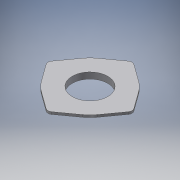
# Autodesk Inventor part: 付け根ロール_サブフレーム_1_3
Saved by Autodesk Inventor 2018 (Build 220112000, 112)
## iProperties
Created: 2016-05-02
Part Number: 付け根ロール_サブフレーム_1_3
Material: アルミニウム 2014-T4
Document SubType Name: Modeling
Designer: hiroaki
Density: 2.8 g/cm^3
Appearance: サテン
Mass: 6.12812 g
Surface Area: 34.4322 cm^2
Volume: 2.18861 cm^3
Author: hiroaki
Autodesk Inventor part; units mm, degrees
ref_plane "YZ Plane" through (0, 0, 0) normal (1, 0, 0) x (0, 1, 0)
ref_plane "XZ Plane" through (0, 0, 0) normal (0, 1, 0) x (-1, 0, 0)
ref_plane "XY Plane" through (0, 0, 0) normal (0, 0, 1) x (1, 0, 0)
derived "付け根ロール_基礎.ipt"
sketch "スケッチ1" plane through (0, 0, 0) normal (0, 0, 1) x (1, 0, 0)
  circle A0 centre (0, 0) radius 5.05 construction
  circle A1 centre (0, -8.5) radius 1.35 construction
  circle A2 centre (0, -8.5) radius 2.5 construction
  circle A3 centre (-5.6569, -5.6569) radius 1.55 construction
  line L0 (-5.6569, -5.6569) -> (0, 0) construction
  line L1 (0, 0) -> (0, -8.5) construction
  line L2 (-4.835, -8.7241) -> (-7.9022, -7.9022) construction
  line L3 (-7.9022, -7.9022) -> (-8.7241, -4.835) construction
  line L4 (-8.7241, -4.835) -> (-6.4787, -2.5896) construction
  line L5 (-6.4787, -2.5896) -> (-3.4115, -3.4115) construction
  line L6 (-3.4115, -3.4115) -> (-2.5896, -6.4787) construction
  line L7 (-2.5896, -6.4787) -> (-4.835, -8.7241) construction
  circle A4 centre (5.6569, -5.6569) radius 1.55 construction
  line L8 (8.7241, -4.835) -> (7.9022, -7.9022) construction
  line L9 (7.9022, -7.9022) -> (4.835, -8.7241) construction
  line L10 (4.835, -8.7241) -> (2.5896, -6.4787) construction
  line L11 (3.4115, -3.4115) -> (6.4787, -2.5896) construction
  line L12 (2.5896, -6.4787) -> (3.4115, -3.4115) construction
  line L13 (6.4787, -2.5896) -> (8.7241, -4.835) construction
  circle A5 centre (8.5, 0) radius 2.5 construction
  circle A6 centre (8.5, 0) radius 1.35 construction
  circle A7 centre (5.6569, 5.6569) radius 1.55 construction
  line L14 (4.835, 8.7241) -> (7.9022, 7.9022) construction
  line L15 (7.9022, 7.9022) -> (8.7241, 4.835) construction
  line L16 (8.7241, 4.835) -> (6.4787, 2.5896) construction
  line L17 (3.4115, 3.4115) -> (2.5896, 6.4787) construction
  line L18 (6.4787, 2.5896) -> (3.4115, 3.4115) construction
  line L19 (2.5896, 6.4787) -> (4.835, 8.7241) construction
  circle A8 centre (0, 8.5) radius 2.5 construction
  circle A9 centre (0, 8.5) radius 1.35 construction
  circle A10 centre (-5.6569, 5.6569) radius 1.55 construction
  line L20 (-8.7241, 4.835) -> (-7.9022, 7.9022) construction
  line L21 (-7.9022, 7.9022) -> (-4.835, 8.7241) construction
  line L22 (-4.835, 8.7241) -> (-2.5896, 6.4787) construction
  line L23 (-3.4115, 3.4115) -> (-6.4787, 2.5896) construction
  line L24 (-2.5896, 6.4787) -> (-3.4115, 3.4115) construction
  line L25 (-6.4787, 2.5896) -> (-8.7241, 4.835) construction
  circle A11 centre (-8.5, 0) radius 2.5 construction
  circle A12 centre (-8.5, 0) radius 1.35 construction
  circle A13 centre (0, 0) radius 12.45 construction
  circle A14 centre (0, 0) radius 21 construction
  circle A15 centre (0, 24.25) radius 3.25 construction
  circle A16 centre (0, 24.25) radius 1.05
  circle A17 centre (-24.25, 0) radius 1.05
  circle A18 centre (0, -24.25) radius 1.05
  circle A19 centre (24.25, 0) radius 1.05
  circle A20 centre (0, 0) radius 21.05 construction
  circle A21 centre (0, 0) radius 27.1368 construction
  circle A22 centre (0, 24.25) radius 2.8868 construction
  line L26 (2.5, 25.6934) -> (2.5, 22.8066) construction
  line L27 (2.5, 22.8066) -> (0, 21.3632) construction
  line L28 (0, 21.3632) -> (-2.5, 22.8066) construction
  line L29 (-2.5, 22.8066) -> (-2.5, 25.6934) construction
  line L30 (-2.5, 25.6934) -> (0, 27.1368) construction
  line L31 (0, 27.1368) -> (2.5, 25.6934) construction
  circle A23 centre (0, 0) radius 11.45
  circle A24 centre (0, 0) radius 22.55 construction
  arc A25 (-13.1973, 18.2848) -> (-18.2848, 13.1973) centre (0, 0) ccw
  line L32 (-13.1973, 18.2848) -> (-1.6895, 26.5907)
  arc A26 (1.6895, 26.5907) -> (-1.6895, 26.5907) centre (0, 24.25) ccw
  line L33 (1.6895, 26.5907) -> (13.1973, 18.2848)
  line L34 (0, 0) -> (0, 24.25) construction
  line L35 (0, 0) -> (8.5, 0) construction
  line L36 (-18.2848, 13.1973) -> (-26.5907, 1.6895)
  arc A27 (-26.5907, 1.6895) -> (-26.5907, -1.6895) centre (-24.25, 0) ccw
  line L37 (-26.5907, -1.6895) -> (-18.2848, -13.1973)
  arc A28 (-18.2848, -13.1973) -> (-13.1973, -18.2848) centre (0, 0) ccw
  line L38 (-13.1973, -18.2848) -> (-1.6895, -26.5907)
  arc A29 (-1.6895, -26.5907) -> (1.6895, -26.5907) centre (0, -24.25) ccw
  line L39 (1.6895, -26.5907) -> (13.1973, -18.2848)
  arc A30 (18.2848, 13.1973) -> (13.1973, 18.2848) centre (0, 0) ccw
  arc A31 (26.5907, -1.6895) -> (26.5907, 1.6895) centre (24.25, 0) ccw
  line L40 (26.5907, 1.6895) -> (18.2848, 13.1973)
  line L41 (26.5907, -1.6895) -> (18.2848, -13.1973)
  arc A32 (13.1973, -18.2848) -> (18.2848, -13.1973) centre (0, 0) ccw
  line L42 (2.75, 25.8377) -> (2.75, 22.6623)
  line L43 (2.75, 22.6623) -> (0, 21.0746)
  line L44 (0, 21.0746) -> (-2.75, 22.6623)
  line L45 (-2.75, 22.6623) -> (-2.75, 25.8377)
  line L46 (-2.75, 25.8377) -> (0, 27.4254)
  line L47 (0, 27.4254) -> (2.75, 25.8377)
  circle A33 centre (24.25, 0) radius 1.55
  circle A34 centre (0, 24.25) radius 1.55
  circle A35 centre (-24.25, 0) radius 1.55
  circle A36 centre (0, -24.25) radius 1.55
  dimension "d8" = 0.05
  dimension "d10" = 5
  dimension "d13" = 1
  dimension "d16" = 42.1
  dimension "d27" = 1.5
  dimension "d38" = 3.1
  dimension "d41" = 360
  measures "d8" radial gap between concentric circles of A20 A14
  measures "d10" distance between parallel lines of L26 L29
  measures "d13" radial gap between concentric circles of A13 A23
  measures "d16" diameter of A20
  measures "d27" radial gap between concentric circles of A24 A20
  measures "d38" diameter of A33
extrude "押し出し1" add sketch "スケッチ1" along normal blind 1.5 contours L32 L45 L44 L43 L42 L33 A30 L40 A31 L41 A32 L39 A29 L38 A28 L37 A27 L36 A25 | L32 L46 A26 L47 L33 L42 L43 L44 L45 | L32 A26 L46 | A26 L33 L47
sketch "スケッチ7" plane through (0, 24.25, 0) normal (0, 0, -1) x (-1, 0, 0)
  circle A0 centre (0, -24.25) radius 11.45 projected
  arc A1 (13.1973, -42.5348) -> (18.2848, -37.4473) centre (0, -24.25) ccw projected
  circle A2 centre (0, -24.25) radius 12.45
  dimension "d35" = 24.9
  constraints: 1 centre point, 1 coincident
  measures "d35" diameter of A2
extrude "押し出し6" add sketch "スケッチ7" along normal blind 2.5
sketch "スケッチ8" plane through (0, 24.25, 0) normal (0, 0, -1) x (-1, 0, 0)
  circle A0 centre (0, 0) radius 1.55 projected
  circle A1 centre (0, 0) radius 1.55
  circle A2 centre (24.25, -24.25) radius 1.55 projected
  circle A3 centre (24.25, -24.25) radius 1.55
  circle A4 centre (0, -48.5) radius 1.55 projected
  circle A5 centre (0, -48.5) radius 1.55
  circle A6 centre (-24.25, -24.25) radius 1.55 projected
  circle A7 centre (-24.25, -24.25) radius 1.55
  point P0 (0, -24.25)
  constraints: 4 centre point, 4 coincident
extrude "押し出し7" add sketch "スケッチ8" against normal up to surface (1.5 mm away)
